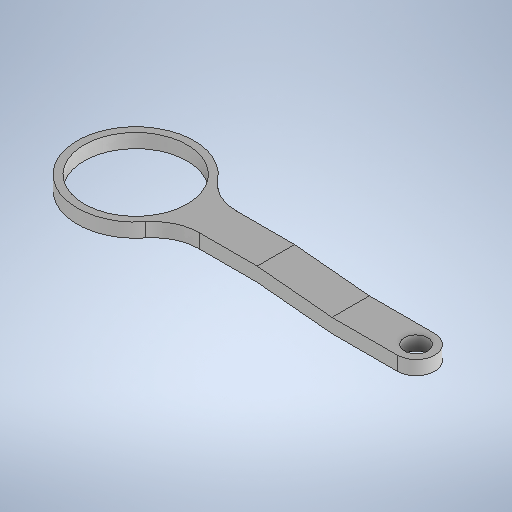
# Autodesk Inventor part: 15B
Saved by Autodesk Inventor 2025.1 (Build 291241000, 241)
## iProperties
Created: 2024-09-17
Part Number: 15B
Material: Generisch
Document SubType Name: Modeling
Designer: ffogue
Density: 1 g/cm^3
Appearance: Vorgabe
Author: ffogue
Autodesk Inventor part; units mm, degrees
ref_plane "YZ Plane" through (0, 0, 0) normal (1, 0, 0) x (0, 1, 0)
ref_plane "XY Plane" through (0, 0, 0) normal (0, 0, 1) x (1, 0, 0)
sketch "Sketch1" plane through (0, 0, 0) normal (0, 0, 1) x (1, 0, 0)
  arc A0 (9.7855, 7.7778) -> (9.7855, -7.7778) centre (0, 0) ccw
  circle A1 centre (0, 0) radius 11
  arc A2 (60, -4) -> (60, 4) centre (60, 0) ccw
  line L0 (60, 4) -> (17.6139, 4) construction
  line L1 (60, -4) -> (17.6139, -4) construction
  arc A3 (17.6139, -4) -> (9.7855, -7.7778) centre (17.6139, -14) ccw
  arc A4 (9.7855, 7.7778) -> (17.6139, 4) centre (17.6139, 14) ccw
  line L2 (30, 4) -> (30, -4) construction
  line L3 (17.6139, -4) -> (17.6139, 4)
  point P0 (11.8427, 4)
  point P1 (11.8427, -4)
  point P2 (-12.5, 0)
  point P3 (30, 0)
  dimension "d0" = 25
  dimension "d1" = 22
  dimension "d2" = 4
  dimension "d3" = 10
  dimension "d4" = 60
  dimension "d17" = 42.5
  constraints: 11 point on circle, 8 end point, 6 tangent, 5 centre point, 4 point on line, 2 coincident, 1 equal radius, 1 horizontal, 1 horizontal alignment, 1 midpoint, 1 perpendicular, 1 vertical, 1 vertical alignment
  measures "d0" diameter of A0
  measures "d1" diameter of A1
  measures "d2" radius of A2
  measures "d3" radius of A3
  measures "d4" distance of A2.centre point (0, 0)
  measures "d17" distance of point (-12.5, 0) point (30, 0)
extrude "Extrusion1" add sketch "Sketch1" against normal blind 3
ref_plane "Work Plane3" through (0, 0, 0) normal (0, 1, 0) x (-1, 0, 0)
sketch "Sketch7" plane through (0, 0, 0) normal (0, 1, 0) x (-1, 0, 0)
  line L0 (-17.6139, 0) -> (-17.6139, -3) projected
  line L1 (-17.6139, -3) -> (-30, -3)
  line L2 (-30, -3) -> (-46, -4.5)
  line L3 (-46, -4.5) -> (-60, -4.5)
  line L4 (-60, -4.5) -> (-60, -1.5)
  line L5 (-60, -1.5) -> (-46, -1.5)
  line L6 (-46, -1.5) -> (-30, 0)
  line L7 (-30, 0) -> (-17.6139, 0)
  line L8 (-17.6139, -3) -> (-17.6139, 0)
  point P0 (0, 0)
  point P1 (-60, -3)
  dimension "d19" = 1.5
  dimension "d20" = 14
  dimension "d21" = 60
  dimension "d22" = 3
  constraints: 16 end point, 3 parallel, 2 perpendicular, 1 collinear, 1 horizontal, 1 midpoint, 1 vertical alignment
  measures "d19" distance from line of L4.end L7
  measures "d20" distance of L4.end L5.end
  measures "d21" horizontal distance of point (-60, -3) point (0, 0)
  measures "d22" distance of L3.end L4.end
extrude "Extrusion3" add sketch "Sketch7" along normal mid plane 8
sketch "Sketch8" plane through (46, 4, -1.5) normal (0, 0, 1) x (1, 0, 0)
  line L0 (14, -8) -> (14, 0) projected
  arc A0 (14, -8) -> (14, 0) centre (14, -4) ccw
  point P0 (-46, -4)
  dimension "d25" = 4
  constraints: 2 point on circle, 1 centre point
  measures "d25" radius of A0
extrude "Extrusion4" add sketch "Sketch8" against normal up to surface (3 mm away)
sketch "Sketch9" plane through (46, -4, -1.5) normal (0, 0, 1) x (1, 0, 0)
  arc A0 (14, 0) -> (14, 8) centre (14, 4) ccw projected
  point P0 (-46, 4)
  constraints: 1 coincident
hole "Hole1" at (60, 0, -1.5) direction (0, 0, -1) diameter 5 depth 3
body "Solid1"
